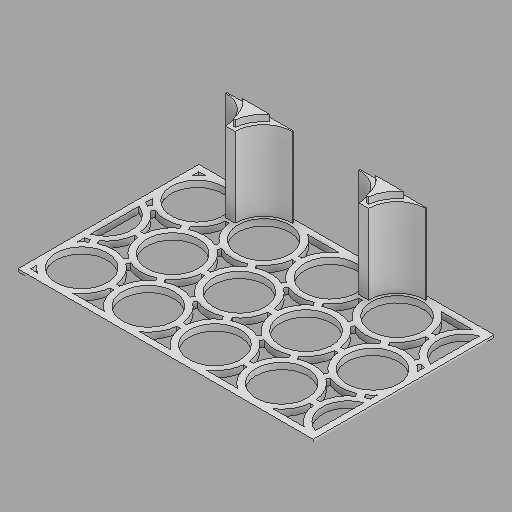
# Autodesk Inventor part: TubeHolder
Saved by Autodesk Inventor 2025 (Build 290162010, 162A)
## iProperties
Created: 2025-03-06
Part Number: TubeHolder
Material: Generic
Document SubType Name: Modeling
Designer: schanen
Density: 1 g/cm^3
Appearance: Default
Author: schanen
Autodesk Inventor part; units mm, degrees
ref_plane "YZ Plane" through (0, 0, 0) normal (1, 0, 0) x (0, 1, 0)
ref_plane "XZ Plane" through (0, 0, 0) normal (0, 1, 0) x (-1, 0, 0)
ref_plane "XY Plane" through (0, 0, 0) normal (0, 0, 1) x (1, 0, 0)
sketch "Sketch1" plane through (0, 0, 0) normal (0, 1, 0) x (-1, 0, 0)
  line L0 (-46.5, 28.5) -> (46.5, 28.5)
  line L1 (46.5, 28.5) -> (46.5, -28.5)
  line L2 (46.5, -28.5) -> (-46.5, -28.5)
  line L3 (-46.5, -28.5) -> (-46.5, 28.5)
  line L4 (-46.5, 28.5) -> (46.5, -28.5) construction
  line L5 (46.5, 28.5) -> (-46.5, -28.5) construction
  circle A0 centre (36.75, -18.1865) radius 8.1
  line L6 (36.75, -18.1865) -> (23.7803, 4.2776)
  circle A1 centre (26.25, 0) radius 8.1
  circle A2 centre (15.75, 18.1865) radius 8.1
  circle A3 centre (15.75, -18.1865) radius 8.1
  circle A4 centre (5.25, 0) radius 8.1
  circle A5 centre (-5.25, 18.1865) radius 8.1
  circle A6 centre (57.75, -18.1865) radius 8.1
  circle A7 centre (47.25, 0) radius 8.1
  circle A8 centre (36.75, 18.1865) radius 8.1
  circle A9 centre (-5.25, -18.1865) radius 8.1
  circle A10 centre (-15.75, 0) radius 8.1
  circle A11 centre (-26.25, 18.1865) radius 8.1
  circle A12 centre (78.75, -18.1865) radius 8.1
  circle A13 centre (68.25, 0) radius 8.1
  circle A14 centre (57.75, 18.1865) radius 8.1
  circle A15 centre (-26.25, -18.1865) radius 8.1
  circle A16 centre (-36.75, 0) radius 8.1
  circle A17 centre (-47.25, 18.1865) radius 8.1
  circle A18 centre (36.75, -18.1865) radius 10
  circle A19 centre (26.25, 0) radius 10
  circle A20 centre (15.75, 18.1865) radius 10
  circle A21 centre (15.75, -18.1865) radius 10
  circle A22 centre (5.25, 0) radius 10
  circle A23 centre (-5.25, 18.1865) radius 10
  circle A24 centre (57.75, -18.1865) radius 10
  circle A25 centre (47.25, 0) radius 10
  circle A26 centre (36.75, 18.1865) radius 10
  circle A27 centre (-5.25, -18.1865) radius 10
  circle A28 centre (-15.75, 0) radius 10
  circle A29 centre (-26.25, 18.1865) radius 10
  circle A30 centre (78.75, -18.1865) radius 10
  circle A31 centre (68.25, 0) radius 10
  circle A32 centre (57.75, 18.1865) radius 10
  circle A33 centre (-26.25, -18.1865) radius 10
  circle A34 centre (-36.75, 0) radius 10
  circle A35 centre (-47.25, 18.1865) radius 10
  line L7 (-44.5, 26.5) -> (44.5, 26.5)
  line L8 (44.5, 26.5) -> (44.5, -26.5)
  line L9 (44.5, -26.5) -> (-44.5, -26.5)
  line L10 (-44.5, -26.5) -> (-44.5, 26.5)
  line L11 (-44.5, 26.5) -> (44.5, -26.5) construction
  line L12 (44.5, 26.5) -> (-44.5, -26.5) construction
  circle A36 centre (99.75, -18.1865) radius 8.1
  circle A37 centre (89.25, 0) radius 8.1
  circle A38 centre (78.75, 18.1865) radius 8.1
  circle A39 centre (-47.25, -18.1865) radius 8.1
  circle A40 centre (-57.75, 0) radius 8.1
  circle A41 centre (-68.25, 18.1865) radius 8.1
  circle A42 centre (99.75, -18.1865) radius 10
  circle A43 centre (89.25, 0) radius 10
  circle A44 centre (78.75, 18.1865) radius 10
  circle A45 centre (-47.25, -18.1865) radius 10
  circle A46 centre (-57.75, 0) radius 10
  circle A47 centre (-68.25, 18.1865) radius 10
  point P0 (0, 0)
  point P1 (44.5, -24.5061)
  point P2 (42.3075, -26.5)
  point P3 (42.3075, 26.5)
  point P4 (44.5, 24.5061)
  point P5 (44.5, -11.8669)
  point P6 (31.1925, -26.5)
  point P7 (21.3075, -26.5)
  point P8 (10.1925, -26.5)
  point P9 (0.3075, -26.5)
  point P10 (-10.8075, -26.5)
  point P11 (-20.6925, -26.5)
  point P12 (-31.8075, -26.5)
  point P13 (-44.5, -6.3196)
  point P14 (-44.5, 6.3196)
  point P15 (-31.8075, 26.5)
  point P16 (-20.6925, 26.5)
  point P17 (-10.8075, 26.5)
  point P18 (0.3075, 26.5)
  point P19 (10.1925, 26.5)
  point P20 (21.3075, 26.5)
  point P21 (31.1925, 26.5)
  point P22 (44.5, 11.8669)
  point P23 (-44.5, 25.8054)
  point P24 (-44.5, 10.5676)
  point P25 (-44.5, 8.5721)
  point P26 (-41.6925, 26.5)
  point P27 (-44.5, -8.5721)
  point P28 (-44.5, -10.5676)
  point P29 (-44.5, -25.8054)
  point P30 (-41.6925, -26.5)
  point P31 (44.5, -9.6144)
  point P32 (44.5, -7.6189)
  point P33 (44.5, 7.6189)
  point P34 (44.5, 9.6144)
  dimension "d0" = 93
  dimension "d1" = 57
  dimension "d2" = 16.2
  dimension "d3" = 60
  dimension "d6" = 21
  dimension "d9" = 21
  dimension "d12" = 10.3135
  dimension "d13" = 9.75
  dimension "d14" = 36.3731
  dimension "d15" = 20
  dimension "d18" = 21
  dimension "d21" = 21
  dimension "d24" = 2
  dimension "d25" = 2
  constraints: 48 centre point, 26 end point, 4 horizontal, 4 midpoint, 4 parallel, 2 perpendicular, 1 coincident, 94 other
  measures "d0" distance of L1.end L2.end
  measures "d1" distance of L0.end L1.end
  measures "d2" diameter of A0
  measures "d3" angle of L2 L6
  measures "d6" distance of L6.start A1.centre
  measures "d9" distance of L6.start A3.centre
  measures "d12" distance from line of L2 L6.start
  measures "d13" distance from line of L1 L6.start
  measures "d14" distance of A11.centre A15.centre
  measures "d15" diameter of A18
  measures "d18" distance of A18.centre A19.centre
  measures "d21" distance of A18.centre A21.centre
  measures "d24" distance between parallel lines of L2 L9
  measures "d25" distance between parallel lines of L1 L8
extrude "Extrusion1" add sketch "Sketch1" along normal blind 2 contours L0 L1 A26 L8 L7 A20 A23 A29 A35 L3 | A35 L7 L10 A17 L3 | L1 A26 L8 A8 | A17 L10 L3 | A35 L10 A17 L7 | A35 L10 A34 L3 | L3 A17 L10 A35 | L1 A25 L8 A26 | L8 A8 A26 L7 | L7 A29 | A29 L7 | A34 L10 A16 L3 | L1 A7 L8 A25 | L7 A26 | A34 L10 A45 L3 | A34 L10 A16 | L1 A7 L8 | L8 A7 A25 | L7 A23 | A23 L7 | A45 L10 A39 L3 | L1 A25 L8 A7 | L1 A18 L8 A25 | L7 A20 | A20 L7 | A39 L10 L3 | A45 L9 L10 A39 | A45 L9 A33 A27 A21 A18 L8 L1 L2 L3 | L3 A39 L10 L9 A45 | L1 A18 L8 A0 | L8 A0 L6 A18 | L6 A0 L8 A18 L9 | L9 A33 | A33 L9 | L9 A18 | L9 A21 | A21 L9 | L9 A27 | A27 L9 | A19 | A22 | A28
sketch "Sketch3" plane through (0, 2, 0) normal (0, 1, 0) x (1, 0, 0)
  circle A0 centre (-36.75, 18.1865) radius 8.1 projected
  circle A1 centre (-26.25, 0) radius 8.1 projected
  line L0 (-36.75, 18.1865) -> (-26.25, 0)
  circle A2 centre (-15.75, 18.1865) radius 8.1 projected
  line L1 (-36.75, 18.1865) -> (-15.75, 18.1865)
  line L2 (-33.597, 10.7254) -> (-31.135, 6.4611)
  line L3 (-31.865, 11.7254) -> (-29.403, 7.4611)
  arc A3 (-33.597, 10.7254) -> (-31.865, 11.7254) centre (-36.75, 18.1865) ccw
  arc A4 (-29.403, 7.4611) -> (-31.135, 6.4611) centre (-26.25, 0) ccw
  point P0 (0, 0)
  dimension "d28" = 1
  dimension "d29" = 1
  constraints: 8 end point, 8 point on circle, 2 centre point, 2 coincident, 2 parallel, 1 horizontal
  measures "d28" distance between parallel lines of L0 L2
  measures "d29" distance between parallel lines of L3 L0
extrude "Extrusion2" add sketch "Sketch3" against normal up to surface (2 mm away) contours A0 L0 A1 L2 | L3 A1 L0 A0
pattern_linear "Rectangular Pattern1" count 2 spacing 21 along (0.5, 0, 0.8660254) count 4 spacing 21 along (1, 0, 0) of "Extrusion2"
mirror "Mirror1" about plane through (0, 0, 0) normal (0, 0, 1) of "Extrusion2", "Rectangular Pattern1"
sketch "Sketch5" plane through (0, 2, 0) normal (0, 1, 0) x (1, 0, 0)
  line L0 (-28.712, 19.1865) -> (-23.788, 19.1865)
  circle A0 centre (-15.75, 18.1865) radius 8.1 projected
  circle A1 centre (-36.75, 18.1865) radius 8.1 projected
  line L1 (-28.712, 17.1865) -> (-23.788, 17.1865)
  arc A2 (-28.712, 17.1865) -> (-28.712, 19.1865) centre (-36.75, 18.1865) ccw
  arc A3 (-23.788, 19.1865) -> (-23.788, 17.1865) centre (-15.75, 18.1865) ccw
  point P0 (0, 0)
  dimension "d38" = 1
  dimension "d39" = 1
  constraints: 8 point on circle, 4 end point, 2 centre point, 2 coincident, 2 horizontal
  measures "d38" distance from line of A1.centre L1
  measures "d39" distance from line of A1.centre L0
extrude "Extrusion3" add sketch "Sketch5" against normal up to surface (2 mm away) contours L0 A0 L1 A1
pattern_linear "Rectangular Pattern2" count 2 spacing 36.3731 along (0, 0, 1) count 4 spacing 21 along (1, 0, 0) of "Extrusion3"
sketch "Sketch6" plane through (0, 2, 0) normal (0, 1, 0) x (1, 0, 0)
  circle A0 centre (36.75, 0) radius 8.1 projected
  line L0 (28.712, 1) -> (23.788, 1)
  circle A1 centre (15.75, 0) radius 8.1 projected
  line L1 (28.712, -1) -> (23.788, -1)
  circle A2 centre (15.75, 0) radius 8.1 projected
  arc A3 (28.712, 1) -> (28.712, -1) centre (36.75, 0) ccw
  arc A4 (23.788, -1) -> (23.788, 1) centre (15.75, 0) ccw
  point P0 (0, 0)
  dimension "d48" = 1
  dimension "d49" = 1
  constraints: 8 point on circle, 4 end point, 2 centre point, 2 coincident, 2 horizontal, 1 point on line, 2 other
  measures "d48" distance from line of A0.centre L1
  measures "d49" distance from line of A0.centre L0
extrude "Extrusion4" add sketch "Sketch6" against normal up to surface (2 mm away) contours A0 L1 A1 L0
pattern_linear "Rectangular Pattern3" count 4 spacing 21 along (-1, 0, 0) of "Extrusion4"
sketch "Sketch7" plane through (0, 2, 0) normal (0, 1, 0) x (1, 0, 0)
  circle A0 centre (-36.75, 18.1865) radius 8.1 projected
  circle A1 centre (-36.75, -18.1865) radius 8.1 projected
  line L0 (-36.75, 18.1865) -> (-36.75, -18.1865) construction
  line L1 (-32.6411, 9.0697) -> (-32.091, 8.1168) projected
  line L2 (-30.3589, 9.1168) -> (-30.909, 10.0697) projected
  line L3 (-32.6411, -9.0697) -> (-32.091, -8.1168) projected
  line L4 (-30.3589, -9.1168) -> (-30.909, -10.0697) projected
  line L5 (-40.8589, 9.0697) -> (-41.409, 8.1168)
  line L6 (-43.1411, 9.1168) -> (-42.591, 10.0697)
  line L7 (-40.8589, -9.0697) -> (-41.409, -8.1168)
  line L8 (-43.1411, -9.1168) -> (-42.591, -10.0697)
  arc A2 (-44.5, -7.6189) -> (-44.5, 7.6189) centre (-47.25, 0) ccw projected
  arc A3 (-41.409, 8.1168) -> (-43.1411, 9.1168) centre (-47.25, 0) ccw
  arc A4 (-42.591, 10.0697) -> (-40.8589, 9.0697) centre (-36.75, 18.1865) ccw
  arc A5 (-40.8589, -9.0697) -> (-42.591, -10.0697) centre (-36.75, -18.1865) ccw
  arc A6 (-43.1411, -9.1168) -> (-41.409, -8.1168) centre (-47.25, 0) ccw
  point P0 (0, 0)
  constraints: 10 end point, 8 point on circle, 8 symmetric about line, 4 centre point, 4 coincident, 1 vertical
extrude "Extrusion5" add sketch "Sketch7" against normal up to surface (2 mm away) contours L5 A3 L6 A4 | A5 L8 A6 L7
sketch "Sketch8" plane through (0, 2, 0) normal (0, 1, 0) x (1, 0, 0)
  circle A0 centre (-36.75, 18.1865) radius 8.1 projected
  circle A1 centre (-15.75, 18.1865) radius 8.1 projected
  line L0 (-36.75, 18.1865) -> (-15.75, 18.1865)
  line L1 (-36.75, 18.1865) -> (-36.75, 27.5)
  line L2 (46.5, 28.5) -> (-46.5, 28.5) projected
  line L3 (-15.75, 18.1865) -> (-15.75, 27.5)
  circle A2 centre (-36.75, 18.1865) radius 9
  circle A3 centre (-15.75, 18.1865) radius 9
  line L4 (-36.75, 27.5) -> (-15.75, 27.5)
  line L5 (-31.1925, 26.5) -> (-21.3075, 26.5) projected
  arc A4 (-26.8001, 19.1865) -> (-31.1925, 26.5) centre (-36.75, 18.1865) ccw projected
  line L6 (-25.6999, 19.1865) -> (-26.8001, 19.1865) projected
  arc A5 (-21.3075, 26.5) -> (-25.6999, 19.1865) centre (-15.75, 18.1865) ccw projected
  point P0 (0, 0)
  point P1 (-36.75, 27.1865)
  point P2 (-27.75, 18.1865)
  point P3 (-24.75, 18.1865)
  point P4 (-15.75, 27.1865)
  dimension "d57" = 1
  dimension "d58" = 18
  dimension "d59" = 18
  constraints: 8 end point, 2 centre point, 2 coincident, 2 horizontal, 2 vertical
  measures "d57" distance from line of L2 L1.end
  measures "d58" diameter of A2
  measures "d59" diameter of A3
extrude "Extrusion6" add sketch "Sketch8" along normal blind 25 contours A2 L1 L4 L3 A3 L0 | L5 A5 L6 A4
pattern_linear "Rectangular Pattern4" count 2 spacing 42 along (1, 0, 0) of "Extrusion6"
sketch "Sketch13" plane through (5.25, 27, -27.5) normal (0, 1, 0) x (1, 0, 0)
  arc A0 (9.9499, -8.3135) -> (5.5575, -1) centre (0, -9.3135) ccw projected
  arc A1 (15.4425, -1) -> (11.0501, -8.3135) centre (21, -9.3135) ccw projected
  line L0 (5.5575, -1) -> (15.4425, -1) projected
  arc A2 (-26.5575, -1) -> (-30.9499, -8.3135) centre (-21, -9.3135) ccw projected
  arc A3 (-32.0501, -8.3135) -> (-36.4425, -1) centre (-42, -9.3135) ccw projected
  line L1 (-21, 0) -> (-42, 0) construction
  line L2 (-36.4425, -1) -> (-26.5575, -1) projected
  line L3 (11.0501, -8.3135) -> (9.9499, -8.3135) projected
  line L4 (-30.9499, -8.3135) -> (-32.0501, -8.3135) projected
  arc A4 (-27.1816, -1.2) -> (-31.1292, -8.1135) centre (-21, -9.3135) ccw
  line L5 (-31.1292, -8.1135) -> (-31.8708, -8.1135)
  arc A5 (-31.8708, -8.1135) -> (-35.8184, -1.2) centre (-42, -9.3135) ccw
  line L6 (-35.8184, -1.2) -> (-27.1816, -1.2)
  line L7 (-21, -0.1998) -> (-42, -0.1998)
  arc A6 (14.8184, -1.2) -> (10.8708, -8.1135) centre (21, -9.3135) ccw
  line L8 (10.8708, -8.1135) -> (10.1292, -8.1135)
  arc A7 (10.1292, -8.1135) -> (6.1816, -1.2) centre (0, -9.3135) ccw
  line L9 (6.1816, -1.2) -> (14.8184, -1.2)
  point P0 (-5.25, -27.5)
  dimension "d71" = 0.2
  dimension "d72" = 0.2
  constraints: 10 end point, 8 point on circle, 4 centre point, 1 parallel, 6 other
  measures "d71" distance between parallel lines of L2 L6
  measures "d72" distance between parallel lines of L0 L9
extrude "Extrusion9" add sketch "Sketch13" along normal blind 2 contours A4 L5 A5 L6 | A6 L8 A7 L9
sketch "Sketch14" plane through (0, 2, 0) normal (0, -1, 0) x (1, 0, 0)
  arc A0 (-30.5684, -26.3) -> (-26.6208, -19.3865) centre (-36.75, -18.1865) ccw projected
  line L0 (-25.8792, -19.3865) -> (-26.6208, -19.3865) projected
  arc A1 (-25.8792, -19.3865) -> (-21.9316, -26.3) centre (-15.75, -18.1865) ccw projected
  line L1 (-30.5684, -26.3) -> (-21.9316, -26.3) projected
  arc A2 (11.4316, -26.3) -> (15.3792, -19.3865) centre (5.25, -18.1865) ccw projected
  line L2 (16.1208, -19.3865) -> (15.3792, -19.3865) projected
  arc A3 (16.3001, -19.1865) -> (20.6925, -26.5) centre (26.25, -18.1865) ccw construction
  arc A4 (16.1208, -19.3865) -> (20.0684, -26.3) centre (26.25, -18.1865) ccw projected
  line L3 (11.4316, -26.3) -> (20.0684, -26.3) projected
  point P0 (0, 0)
extrude "Extrusion10" add sketch "Sketch14" along normal up to surface (2 mm away)
fillet "Fillet1" radius 2 4 edges at (0, 0, 28.5) (-46.5, 0, 0) (46.5, 0, 0) (0, 0, -28.5)
equation "\"d12\" = -0.5 * d14 + 0.5 * d1"
equation "\"d18\" = d6"
equation "\"d21\" = d9"
equation "\"d29\" = d28"
equation "\"d44\" = d14"
equation "\"d59\" = d58"
body "Solid1"
